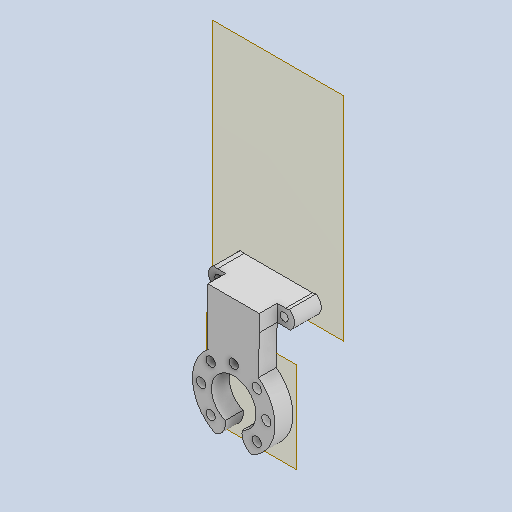
# Autodesk Inventor part: 0904_thigh_2
Saved by Autodesk Inventor 2024.3 (Build 283343000, 343)
## iProperties
Created: 2024-09-04
Part Number: 0904_thigh_2
Material: 일반
Document SubType Name: Modeling
Designer: gretc
Density: 1 g/cm^3
Appearance: 기본값
Author: gretc
Autodesk Inventor part; units mm, degrees
ref_plane "YZ Plane" through (0, 0, 0) normal (1, 0, 0) x (0, 1, 0)
ref_plane "XZ Plane" through (0, 0, 0) normal (0, 1, 0) x (-1, 0, 0)
ref_plane "XY Plane" through (0, 0, 0) normal (0, 0, 1) x (1, 0, 0)
ref_plane "작업 평면1" through (0, 0, 0) normal (0, 0, 1) x (1, 0, 0)
sketch "스케치1" plane through (0, 0, 0) normal (0, 0, 1) x (1, 0, 0)
  line L0 (-15, 14.5) -> (-11.5, 14.5) projected
  line L1 (-15, 14.5) -> (-20.1, 8.5) projected
  line L2 (-20.1, 8.5) -> (-20.1, -44.6) projected
  line L3 (-20.1, -44.6) -> (-15, -50.6) projected
  line L4 (-15, -50.6) -> (15, -50.6) projected
  line L5 (15, -50.6) -> (20.1, -44.6) projected
  line L6 (20.1, -44.6) -> (20.1, 8.5) projected
  line L7 (20.1, 8.5) -> (15, 14.5) projected
  line L8 (11.5, 14.5) -> (15, 14.5) projected
  arc A0 (14.5, 11.5) -> (11.5, 14.5) centre (11.5, 11.5) ccw projected
  line L9 (14.5, -42) -> (14.5, 11.5) projected
  arc A1 (11.5, -45) -> (14.5, -42) centre (11.5, -42) ccw projected
  line L10 (-11.5, -45) -> (11.5, -45) projected
  arc A2 (-14.5, -42) -> (-11.5, -45) centre (-11.5, -42) ccw projected
  line L11 (-14.5, 11.5) -> (-14.5, -42) projected
  arc A3 (-11.5, 14.5) -> (-14.5, 11.5) centre (-11.5, 11.5) ccw projected
  circle A4 centre (17.3, 4) radius 1.35 projected
  circle A5 centre (17.3, -18) radius 1.35 projected
  circle A6 centre (17.3, -40) radius 1.35 projected
  circle A7 centre (11, -47.8) radius 1.35 projected
  circle A8 centre (-17.3, 4) radius 1.35 projected
  circle A9 centre (-17.3, -18) radius 1.35 projected
  circle A10 centre (-17.3, -40) radius 1.35 projected
  circle A11 centre (-11, -47.8) radius 1.35 projected
  circle A12 centre (11, -47.8) radius 3.5
  circle A13 centre (-11, -47.8) radius 3.5
  point P0 (0, 0)
  point P1 (12.709, -44.7456)
  point P2 (-12.709, -44.7456)
  point P3 (-13.1, -50.6)
  point P4 (13.1, -50.6)
  dimension "d0" = 7
  dimension "d1" = 7
  constraints: 2 centre point, 2 coincident
  measures "d0" diameter of A12
  measures "d1" diameter of A13
extrude "돌출1" add sketch "스케치1" along normal blind 9 contours A2 L10 A13 L4 | L10 A12 L4 A13 | L10 A1 A12 L4
ref_plane "작업 평면2" through (0, -75, 9) normal (0, 0, 1) x (-0.0000047, -1, 0)
sketch "스케치2" plane through (0, -75, 9) normal (0, 0, 1) x (-0.0000047, -1, 0)
  circle A0 centre (-7.7782, -7.7782) radius 1.55 projected
  circle A1 centre (7.7782, -7.7782) radius 1.55 projected
  circle A2 centre (7.7782, 7.7782) radius 1.55 projected
  circle A3 centre (-7.7782, 7.7782) radius 1.55 projected
  circle A4 centre (0, 0) radius 5 projected
  circle A5 centre (0, 0) radius 13.9 projected
  circle A6 centre (0, 11) radius 1.55 projected
  circle A7 centre (11, 0) radius 1.55 projected
  circle A8 centre (0, -11) radius 1.55 projected
  circle A9 centre (-11, 0) radius 1.55 projected
  arc A10 (-30.0001, 11.4999) -> (-30.2545, 12.7088) centre (-33.0001, 11.4998) ccw projected
  line L0 (-30.0001, 11.4999) -> (-29.9999, -11.5001) projected
  arc A11 (-30.2543, -12.7091) -> (-29.9999, -11.5001) centre (-32.9999, -11.5002) ccw projected
  arc A12 (-30.2543, -12.7091) -> (-24.3999, -13.1001) centre (-27.1999, -11.0001) ccw projected
  line L1 (-24.3999, -13.1001) -> (-24.4001, 13.0999) projected
  arc A13 (-24.4001, 13.0999) -> (-30.2545, 12.7088) centre (-27.2001, 10.9999) ccw projected
  circle A14 centre (-27.1999, -11.0001) radius 1.35 projected
  circle A15 centre (-27.2001, 10.9999) radius 1.35 projected
  line L2 (-24.4, 8.6132) -> (-11, 8.333) projected
  line L3 (-10.6944, -8.7218) -> (-24.4, -8.7218) projected
  line L4 (-24.4, -9.0001) -> (-29, -9.0001) projected
  line L5 (-24.4, 8.5249) -> (-28.629, 8.5249) projected
  line L6 (-24.4, -8.5251) -> (-28.6289, -8.5251) projected
  line L7 (-24.4, 8.6132) -> (-30, 8.6132)
  line L8 (-30.0001, 11.4999) -> (-29.9999, -11.5001) projected
  line L9 (-24.4, -8.7218) -> (-30, -8.7219)
  circle A16 centre (7.7782, 7.7782) radius 5
  circle A17 centre (7.7782, -7.7782) radius 5
  circle A18 centre (0, 0) radius 7.5 projected
  circle A19 centre (0, 0) radius 7.5 projected
  point P0 (-75, -0.0004)
  point P1 (6.9377, 2.8493)
  point P2 (12.4889, 6.1022)
  point P3 (-11.1233, 8.3356)
  point P4 (-30, 8.6132)
  point P5 (-30, -8.7219)
  point P6 (-10.8232, -8.7218)
  point P7 (12.4889, -6.1022)
  point P8 (6.9377, -2.8493)
  dimension "d4" = 10
  dimension "d5" = 10
  constraints: 4 end point, 2 centre point, 2 coincident, 2 point on line, 1 parallel, 1 perpendicular
  measures "d4" diameter of A16
  measures "d5" diameter of A17
extrude "돌출2" add sketch "스케치2" along normal blind 6 contours A16 A18 A5 | A5 A17 A18 | A16 A18 A17 A5 | A5 L3 L1 L2 | L1 L9 L0 L7 picked at (-10.7158, 4.5818)
